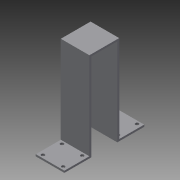
# Autodesk Inventor part: Sheet Metal Arm v2
Saved by Autodesk Inventor 2015 (Build 190159000, 159)
## iProperties
Created: 2015-02-27
Part Number: Sheet Metal Arm v2
Material: Generic
Document SubType Name: Modeling
Designer: pltwe4
Density: 1 g/cm^3
Appearance: Default
Author: pltwe4
Autodesk Inventor part; units mm, degrees
ref_plane "YZ Plane" through (0, 0, 0) normal (1, 0, 0) x (0, 1, 0)
ref_plane "XZ Plane" through (0, 0, 0) normal (0, 1, 0) x (-1, 0, 0)
ref_plane "XY Plane" through (0, 0, 0) normal (0, 0, 1) x (1, 0, 0)
sketch "Sketch1" plane through (0, 0, 0) normal (1, 0, 0) x (0, 1, 0)
  line L0 (0, 67) -> (0, 21.825)
  line L1 (0, 21.825) -> (146.825, 21.825)
  line L2 (146.825, 21.825) -> (146.825, -21.825)
  line L3 (146.825, -21.825) -> (0, -21.825)
  line L4 (0, -21.825) -> (0, -67)
  line L5 (0, -67) -> (3.175, -67)
  line L6 (3.175, -67) -> (3.175, -25)
  line L7 (3.175, -25) -> (150, -25)
  line L8 (150, -25) -> (150, 25)
  line L9 (150, 25) -> (3.175, 25)
  line L10 (3.175, 25) -> (3.175, 67)
  line L11 (3.175, 67) -> (0, 67)
  line L12 (6.6614, 25) -> (6.6614, 21.825) construction
  line L13 (146.825, 0) -> (150, 0) construction
  line L14 (6.6614, -21.825) -> (6.6614, -25) construction
  line L15 (-30, 0) -> (180, 0) construction
  line L16 (106.5396, 7.913) -> (72.5659, 7.913) construction
  line L17 (114.8237, 28.913) -> (65.8343, 28.913) construction
  point P0 (0, 0)
  dimension "d0" = 3.175
  dimension "d2" = 50
  dimension "d3" = 150
  dimension "d4" = 29.738
  dimension "d5" = 21
  dimension "d24" = 42
  constraints: 34 end point, 16 perpendicular, 9 point on line, 2 horizontal, 2 midpoint, 1 vertical, 4 other
  measures "d0" distance of L10.end L0.start
  measures "d2" distance of L7.end L8.end
  measures "d3" distance between parallel lines of L0 L8
  measures "d4" distance between parallel lines of L3 L16
  measures "d5" distance between parallel lines of L16 L17
  measures "d24" distance between parallel lines of L11 L9
extrude "Extrusion1" add sketch "Sketch1" along normal mid plane 48
sketch "Sketch2" plane through (-24, 0, 21.825) normal (0, -1, 0) x (1, 0, 0)
  line L0 (0, 0) -> (0, 45.175) projected
  line L1 (0, 0) -> (48, 0) projected
  line L2 (48, 45.175) -> (48, 0) projected
  line L3 (48, 45.175) -> (0, 45.175) projected
  line L4 (0, -88.825) -> (0, -43.65) projected
  line L5 (0, -88.825) -> (48, -88.825) projected
  line L6 (48, -43.65) -> (48, -88.825) projected
  line L7 (0, -43.65) -> (48, -43.65) projected
  line L8 (0, 0) -> (48, 0) projected
  line L9 (0, 0) -> (0, 45.175) projected
  line L10 (24, 71.975) -> (24, -115.625) projected
  point P0 (24, -21.825)
  point P1 (41, 40.175)
  dimension "d9" = 5
  dimension "d10" = 17
  measures "d9" distance from line of L3 point (41, 40.175)
  measures "d10" distance from line of L10 point (41, 40.175)
hole "Hole1" at (17, 0, 62) direction (0, 1, 0) diameter 5.5 end through all
pattern_linear "Rectangular Pattern1" count 2 spacing 32 along (0, 0, -1) count 2 spacing 34 along (-1, 0, 0) of "Hole1"
mirror "Mirror1" about plane through (0, 0, 0) normal (0, 0, 1) of "Hole1", "Rectangular Pattern1"
body "Solid1"
